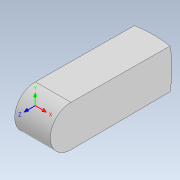
# Autodesk Inventor part: shank
Saved by Autodesk Inventor 2020 (Build 240168000, 168)
## iProperties
Created: 2021-01-07
Part Number: shank
Material: Generic
Document SubType Name: Modeling
Designer: DELL
Density: 1 g/cm^3
Appearance: Default
Author: DELL
Autodesk Inventor part; units mm, degrees
ref_plane "YZ Plane" through (0, 0, 0) normal (1, 0, 0) x (0, 1, 0)
ref_plane "XY Plane" through (0, 0, 0) normal (0, 0, 1) x (1, 0, 0)
ref_plane "UCS1: YZ Plane" through (0, 0, 0) normal (1, 0, 0) x (0, 1, 0)
sketch "Sketch2" plane through (0, 0, 0) normal (1, 0, 0) x (0, 1, 0)
  circle A0 centre (0, 0) radius 26
  line L0 (25, -130) -> (-25, -130)
  line L1 (0, 0) -> (0, -130) construction
  line L2 (-25.9992, -0.2001) -> (-25, -130)
  line L3 (25.9992, -0.2001) -> (25, -130)
  dimension "d1" = 52
  dimension "d3" = 50
  dimension "d25" = 130
  constraints: 8 end point, 2 coincident, 2 point on circle, 1 centre point, 1 horizontal, 1 midpoint, 1 perpendicular, 1 tangent, 1 other
  measures "d1" diameter of A0
  measures "d3" distance of L0.start L0.end
  measures "d25" distance from line of L0 L1.start
extrude "Extrusion1" add sketch "Sketch2" along normal blind 45 contours A0
extrude "Extrusion2" add sketch "Sketch2" against normal blind 45 from surface at 45 contours A0 L3 L0 L2
sketch "Sketch5" plane through (45, -25, -130) normal (0, 0, -1) x (-1, 0, 0)
  circle A0 centre (22.5, 25) radius 10
  line L0 (45, 50) -> (45, 0) projected
  line L1 (45, 50) -> (0, 50) projected
  point P0 (45, 25)
  point P1 (45, 25)
  point P2 (-45, 0)
  point P3 (22.5, 50)
  dimension "d22" = 20
  constraints: 1 centre point, 1 horizontal alignment, 1 midpoint, 1 vertical alignment, 2 other
  measures "d22" diameter of A0
extrude "Extrusion4" cut sketch "Sketch5" against normal blind 60
ref_plane "Work Plane1" through (22.5, 0, 0) normal (-1, 0, 0) x (0, 0, -1)
sketch "Sketch4" plane through (22.5, 0, 0) normal (-1, 0, 0) x (0, 0, -1)
  line L0 (130, -25) -> (130, 25) projected
  arc A0 (123.6932, -40) -> (130, 0) centre (0, 0) ccw
  line L1 (123.6932, -40) -> (130, -40)
  line L2 (130, -40) -> (130, 0)
  line L3 (-62.4, 0) -> (192.4, 0) projected
  line L4 (0, 0) -> (130, 0)
  point P0 (156, -25)
  point P1 (156, 25)
  point P2 (156, -25)
  point P3 (130, -25)
  point P4 (130, 25)
  point P5 (130, 25)
  point P6 (130, -25)
  point P7 (-25, 130)
  point P8 (25, 130)
  dimension "d18" = 40
  constraints: 6 end point, 2 horizontal, 2 point on circle, 1 centre point, 1 coincident, 1 perpendicular, 2 other
  measures "d18" distance between parallel lines of L3 L1
revolve "Revolution1" cut sketch "Sketch4" angle 360 about axis through (22.5, 0, 0) along (0, 0, -1)
body "Solid1"
